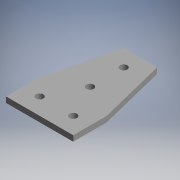
# Autodesk Inventor part: 4341
Saved by Autodesk Inventor 2017.3 (Build 213256000, 256)
## iProperties
Part Number: 4341
Material: Generic
Catalog Web Link: www.cadenas.de
Description: 4141, 4341, 4141-Black, 4341-Black-Joining Plates - 4 Hole Tee Joining Plate
Vendor: 8020
Document SubType Name: Modeling
Designer: partserver
Manufacturer: 8020
Mass: 44.704 g
Surface Area: 169.52 cm^2
Volume: 44.704 cm^3
Density: 1 g/cm^3
Appearance: PSOLRGB-191-191-191
Category: PARTsolutions
Company: 8020
Title: 4341
Author: Cadenas PARTsolutions
Comments: Joining Plates - 4 Hole Tee Joining Plate
PSOL_IDENT_0: {$CADENAS_DATA\23d-libs\8020\inch\joining_plates\4141.prj},176 {VTYP=3D},{NB=4341},{LINA=4341},{NN=4
PSOL_IDENT_1: 141, 4341, 4141-Black, 4341-Black},{DATE=31.07.2020 09:21:18},{GEOMDATE=12.07.2017 12:20:29},{VERSIO
PSOL_IDENT_2: N=},{LINEID=20},{WBVAR=},{WBNUMERIC=}  {NB=4341},{LINA=4341},{KT=DUMMY},{PN=4341},{A=3.000},{B=4.500
PSOL_IDENT_3: },{C=1.500},{F=0.328},{W=.260},{A1=0.7500},{C1=2.250},{C2=0.750},{C3=3.750},{D1=0.250},{COLOR=.75,.7
PSOL_IDENT_4: 5,.75}
NB: 4341
NN: 4141, 4341, 4141-Black, 4341-Black
NT: Joining Plates - 4 Hole Tee Joining Plate
NBSYN: $PN.
LINA: 4341
CATALOG: 80/20
PN: 4341
A: 3
B: 4.5
C: 1.5
W: .260
SUPPLIER: 8020
ARTICLENO: 4341
BOMINFO: 4341
CREATOR: CADENAS GmbH
Autodesk Inventor part; units mm, degrees
ref_plane "YZ Plane" through (0, 0, 0) normal (1, 0, 0) x (0, 1, 0)
ref_plane "XZ Plane" through (0, 0, 0) normal (0, 1, 0) x (-1, 0, 0)
ref_plane "XY Plane" through (0, 0, 0) normal (0, 0, 1) x (1, 0, 0)
sketch "Sketch_1" plane through (0, 0, 0) normal (0, 0, 1) x (1, 0, 0)
  line L0 (-38.1, 38.1) -> (-38.1, 0)
  line L1 (-38.1, 0) -> (38.1, 0)
  line L2 (38.1, 0) -> (38.1, 38.1)
  line L3 (38.1, 38.1) -> (19.05, 114.3)
  line L4 (19.05, 114.3) -> (-19.05, 114.3)
  line L5 (-19.05, 114.3) -> (-38.1, 38.1)
  circle A0 centre (19.05, 19.05) radius 4.1656
  circle A1 centre (0, 57.15) radius 4.1656
  circle A2 centre (0, 95.25) radius 4.1656
  circle A3 centre (-19.05, 19.05) radius 4.1656
  constraints: 12 end point, 4 centre point
extrude "Extrusion1" add sketch "Sketch_1" along normal blind 6.35
body "Solid1"
